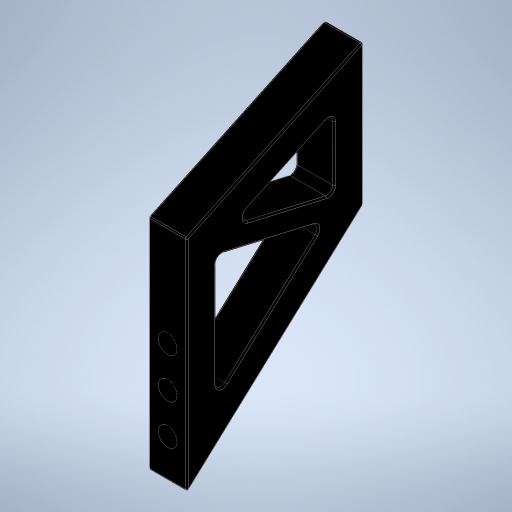
# Autodesk Inventor part: ArmSolderingIron
Saved by Autodesk Inventor 2024 (Build 280153000, 153)
## iProperties
Created: 2023-12-27
Part Number: ArmSolderingIron
Material: Generisch
Document SubType Name: Modeling
Designer: denni
Density: 1 g/cm^3
Appearance: Vorgabe(2)
Author: denni
Autodesk Inventor part; units mm, degrees
ref_plane "YZ Plane" through (0, 0, 0) normal (1, 0, 0) x (0, 1, 0)
ref_plane "XZ Plane" through (0, 0, 0) normal (0, 1, 0) x (-1, 0, 0)
ref_plane "XY Plane" through (0, 0, 0) normal (0, 0, 1) x (1, 0, 0)
sketch "Skizze1" plane through (0, 0, 0) normal (1, 0, 0) x (0, 1, 0)
  line L0 (0, 0) -> (75, 0)
  line L1 (75, 0) -> (103, -60)
  line L2 (103, -60) -> (55, -60)
  line L3 (87.298, -50) -> (68.6314, -10)
  line L4 (68.6314, -10) -> (22.7324, -10)
  line L5 (59.399, -50) -> (87.298, -50)
  line L6 (75, 0) -> (75, -60) construction
  line L7 (55, -60) -> (0, 0)
  line L8 (59.399, -50) -> (22.7324, -10)
  line L9 (68.6314, -10) -> (59.399, -50)
  line L10 (62.991, -50) -> (71.0347, -15.15)
  line L11 (65.0394, -10) -> (56.5295, -46.8696)
  dimension "d1" = 75
  dimension "d3" = 48
  dimension "d6" = 10
  dimension "d32" = 60
  dimension "d33" = 20
  dimension "d42" = 10
  dimension "d43" = 10
  dimension "d44" = 7
  dimension "d45" = 3.5
  constraints: 24 end point, 5 parallel, 5 point on line, 1 horizontal, 1 perpendicular, 1 other
  measures "d1" distance of L0.start L0.end
  measures "d3" distance of L1.end L2.end
  measures "d6" distance between parallel lines of L1 L3
  measures "d32" distance between parallel lines of L2 L0
  measures "d33" distance from line of L6 L2.end
  measures "d42" distance between parallel lines of L7 L8
  measures "d43" distance between parallel lines of L2 L5
  measures "d44" distance between parallel lines of L10 L11
  measures "d45" distance between parallel lines of L10 L9
extrude "Extrusion1" add sketch "Skizze1" along normal blind 13 contours L0 L1 L2 L7 | L10 L5 L9 L3 | L9 L8 L11 L4
sketch "Skizze2" plane through (0, 0, 0) normal (0, 0, 1) x (1, 0, 0)
  line L0 (6.5, 0) -> (6.5, 13.625) construction
  line L1 (6.5, 13.625) -> (6.5, 27.25) construction
  line L2 (6.5, 27.25) -> (6.5, 40.875) construction
  line L3 (0, 0) -> (13, 0) construction
  dimension "d10" = 13.625
  constraints: 6 end point, 4 collinear, 3 coincident, 1 midpoint, 1 perpendicular
  measures "d10" distance of L1.end L2.end
hole "Bohrung1" at (6.5, 40.875, 0) at (6.5, 27.25, 0) at (6.5, 13.625, 0) direction (0, 0, -1) diameter 6.4 depth 6.8
sketch "Skizze4" plane through (0, 55, -60) normal (0, 0, -1) x (-1, 0, 0)
  line L0 (0, 48) -> (-13, 48) construction
  line L1 (-6.5, 48) -> (-6.5, 38) construction
  line L2 (-6.5, 38) -> (-6.5, 10) construction
  line L3 (-6.5, 10) -> (-6.5, 0) construction
  line L4 (0, 0) -> (-13, 0) construction
  point P0 (0, -55)
  dimension "d34" = 10
  constraints: 6 end point, 2 collinear, 2 midpoint, 1 perpendicular
  measures "d34" distance of L1.start L1.end
hole "Bohrung3" at (6.5, 93, -60) at (6.5, 65, -60) direction (0, 0, 1) diameter 5.6 depth 5
fillet "Rundung1" radius 2 7 edges at (6.5, 87.298, -50) (6.5, 16.825, -6.8) (6.5, 22.7324, -10) (6.5, 71.0347, -15.15) (6.5, 62.991, -50) (6.5, 56.5295, -46.8696) (6.5, 65.0394, -10)
fillet "Rundung3" radius 0.5 4 edges at (6.5, 103, -60) (6.5, 55, -60) (6.5, 0, 0) (6.5, 75, 0)
fillet "Rundung4" radius 0.5 26 edges at (0, 55.0186, -59.9577) (0, 78.7174, -60) (0, 102.6366, -59.7686) (0, 88.9013, -29.7886) (0, 74.9502, -0.0783) (0, 37.9091, 0) (0, 0.6789, -0.2987) (13, 55.0186, -59.9577) (13, 78.7174, -60) (13, 102.6366, -59.7686) (13, 88.9013, -29.7886) (13, 74.9502, -0.0783) (13, 37.9091, 0) (13, 0.6789, -0.2987) (0, 25.4481, -11.1947) (0, 64.0903, -10.7549) (0, 44.902, -10) (13, 25.4481, -11.1947) (13, 64.0903, -10.7549) (13, 44.902, -10) (0, 79.73, -33.7829) (0, 85.8446, -49.0744) (0, 74.8314, -50) (13, 79.73, -33.7829) (13, 85.8446, -49.0744) (13, 74.8314, -50)
